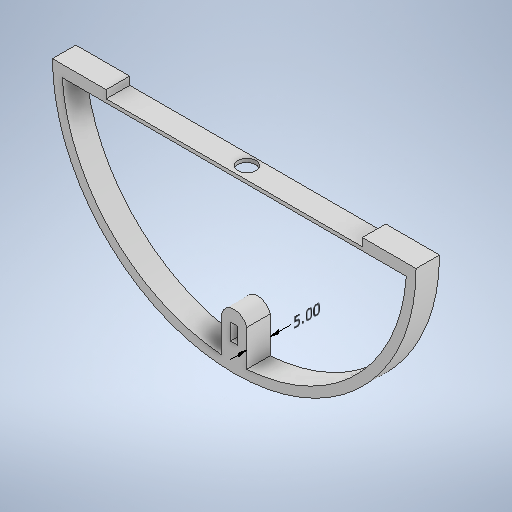
# Autodesk Inventor part: Siding Lock
Saved by Autodesk Inventor 2025 (Build 290162010, 162A)
## iProperties
Created: 2024-06-06
Part Number: Siding Lock
Material: Generic
Document SubType Name: Modeling
Designer: vncnt
Density: 1 g/cm^3
Appearance: Default
Author: vncnt
Autodesk Inventor part; units mm, degrees
ref_plane "YZ Plane" through (0, 0, 0) normal (1, 0, 0) x (0, 1, 0)
ref_plane "XZ Plane" through (0, 0, 0) normal (0, 1, 0) x (-1, 0, 0)
ref_plane "XY Plane" through (0, 0, 0) normal (0, 0, 1) x (1, 0, 0)
sketch "Sketch1" plane through (0, 0, 0) normal (0, 0, 1) x (1, 0, 0)
  arc A0 (37.1972, 10.8951) -> (38.76, 0) centre (0, 0) ccw
  arc A1 (-36.6776, -2.4605) -> (36.6776, -2.4605) centre (0, 0) ccw
  line L0 (-36.76, 0) -> (36.76, 0)
  line L1 (-36.76, 0) -> (37.1972, 0)
  line L2 (36.6776, -2.4605) -> (-36.6776, -2.4605)
  line L3 (-36.76, 0) -> (-38.76, 0)
  line L4 (37.1972, 0) -> (38.76, 0)
  line L5 (0, 0) -> (27.3, 0)
  line L6 (27.3, 0) -> (27.3, -1.7)
  line L7 (27.3, -1.7) -> (0, -1.7)
  line L8 (0, -1.7) -> (0, 0)
  line L9 (-27.3, 0) -> (-27.3, -1.7)
  line L10 (-27.3, -1.7) -> (0, -1.7)
  dimension "d0" = 77.52
  dimension "d1" = 2
  constraints: 22 end point, 5 point on circle, 4 horizontal, 3 parallel, 2 centre point, 2 point on line, 2 symmetric about line, 1 coincident, 1 perpendicular
  measures "d0" diameter of A0
  measures "d1" radial gap between concentric circles of A0 A1
extrude "Extrusion1" add sketch "Sketch1" along normal blind 5 contours L3 L0 L9 L10 L7 L6 L1 L4 A0
sketch "Sketch2" plane through (-27.3, -1.7, 0) normal (0, 1, 0) x (1, 0, 0)
  line L0 (54.6, 0) -> (0, 0) projected
  line L1 (54.6, 0) -> (54.6, -5) projected
  line L2 (0, 0) -> (0, -5) projected
  point P0 (27.3, 0)
  point P1 (27.305, -2.3213)
  dimension "d7" = 2.3213
  dimension "d28" = 27.305
  measures "d7" distance from line of L0 point (27.305, -2.321)
  measures "d28" distance from line of L2 point (27.305, -2.321)
hole "Hole1" at (0.005, -1.7, 2.3213) direction (0, -1, 0) diameter 3.81 depth 2.54
sketch "Sketch3" plane through (0, 0, 5) normal (0, 0, 1) x (1, 0, 0)
  arc A0 (2.6516, -28.9347) -> (-2.75, -29.6637) centre (0, -29.6637) ccw
  line L0 (-0.7992, -29.6638) -> (0.7008, -29.6638)
  line L1 (2.6516, -29.6637) -> (2.6516, -38.4638)
  line L2 (2.6516, -38.4638) -> (-2.75, -38.4638)
  line L3 (-2.75, -38.4638) -> (-2.75, -29.6637)
  line L4 (-0.7992, -29.6638) -> (0.7008, -29.6638)
  line L5 (0.7008, -29.6638) -> (0.7008, -33.1638)
  line L6 (0.7008, -33.1638) -> (-0.7992, -33.1638)
  line L7 (-0.7992, -33.1638) -> (-0.7992, -29.6638)
  line L8 (2.6516, -29.6637) -> (2.6516, -28.9347)
  point P0 (0, 0)
  point P1 (-0.0492, -29.6638)
  point P2 (2.6516, -30.3927)
  dimension "d16" = 5.5
  dimension "d17" = 3.5
  dimension "d18" = 1.5
  dimension "d19" = 0.75
  constraints: 18 end point, 4 parallel, 2 horizontal, 2 perpendicular, 2 point on circle, 1 centre point, 1 midpoint, 1 point on line, 1 vertical
  measures "d16" diameter of A0
  measures "d17" distance of L0.end L5.end
  measures "d18" distance of L5.end L6.end
  measures "d19" distance from line of point (-0.049, -29.664) L5
extrude "Extrusion2" add sketch "Sketch3" against normal up to surface (5 mm away)
body "Solid1"
